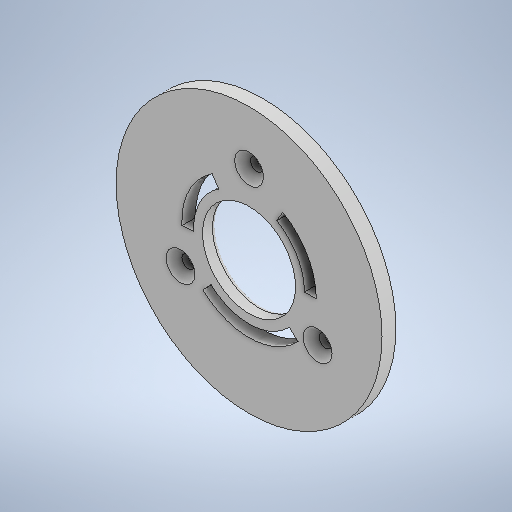
# Autodesk Inventor part: 旋钮帽基座-v0.1.1
Saved by Autodesk Inventor 2025 (Build 290162000, 162)
## iProperties
Created: 2025-05-09
Part Number: 旋钮帽基座-v0.1.1
Material: 常规
Document SubType Name: Modeling
Designer: hawav
Density: 1 g/cm^3
Appearance: 默认
Author: hawav
Autodesk Inventor part; units mm, degrees
ref_plane "YZ Plane" through (0, 0, 0) normal (1, 0, 0) x (0, 1, 0)
ref_plane "XZ Plane" through (0, 0, 0) normal (0, 1, 0) x (-1, 0, 0)
ref_plane "XY Plane" through (0, 0, 0) normal (0, 0, 1) x (1, 0, 0)
sketch "草图1" plane through (0, 0, 0) normal (0, 0, 1) x (1, 0, 0)
  circle A0 centre (0, 0) radius 33.6
  circle A1 centre (0, 0) radius 20
  circle A2 centre (0, 20) radius 1.65
  circle A3 centre (-17.3205, -10) radius 1.65
  circle A4 centre (17.3205, -10) radius 1.65
  circle A5 centre (0, 0) radius 11.75
  circle A6 centre (0, 0) radius 21.65
  line L0 (0, 21.65) -> (0, 33.6)
  circle A7 centre (-5.3894, 27.0942) radius 5.15
  circle A8 centre (-15.3476, 22.9693) radius 5.15
  circle A9 centre (-22.9693, 15.3476) radius 5.15
  circle A10 centre (-27.0942, 5.3894) radius 5.15
  circle A11 centre (-27.0942, -5.3894) radius 5.15
  circle A12 centre (-22.9693, -15.3476) radius 5.15
  circle A13 centre (-15.3476, -22.9693) radius 5.15
  circle A14 centre (-5.3894, -27.0942) radius 5.15
  circle A15 centre (5.3894, -27.0942) radius 5.15
  circle A16 centre (15.3476, -22.9693) radius 5.15
  circle A17 centre (22.9693, -15.3476) radius 5.15
  circle A18 centre (27.0942, -5.3894) radius 5.15
  circle A19 centre (27.0942, 5.3894) radius 5.15
  circle A20 centre (22.9693, 15.3476) radius 5.15
  circle A21 centre (15.3476, 22.9693) radius 5.15
  circle A22 centre (5.3894, 27.0942) radius 5.15
  line L1 (0, 0) -> (0.3894, -13.9946)
  line L2 (0.3894, -13.9946) -> (0.4728, -16.9934)
  arc A23 (0.4728, -16.9934) -> (12.3505, -11.6818) centre (0, 0) ccw
  line L3 (0, 0) -> (12.3505, -11.6818) construction
  line L4 (0, 0) -> (0.4728, -16.9934) construction
  arc A24 (17, 0) -> (8.5, 14.7224) centre (0, 0) ccw
  line L5 (0, 0) -> (8.5, 14.7224) construction
  line L6 (0, 0) -> (17, 0) construction
  arc A25 (0.3894, -13.9946) -> (10.171, -9.6203) centre (0, 0) ccw
  line L7 (0, 0) -> (10.171, -9.6203) construction
  line L8 (0, 0) -> (0.3894, -13.9946) construction
  arc A26 (14, 0) -> (7, 12.1244) centre (0, 0) ccw
  line L9 (7, 12.1244) -> (8.5, 14.7224)
  line L10 (17, 0) -> (14, 0)
  line L11 (12.3505, -11.6818) -> (10.171, -9.6203)
  line L12 (0.4728, -16.9934) -> (0.3894, -13.9946)
  arc A27 (-11.6818, -12.3505) -> (0.4728, -16.9934) centre (0, 0) ccw
  arc A28 (-9.3055, 14.227) -> (-16.9737, -0.9452) centre (0, 0) ccw
  line L13 (0, 0) -> (-9.3055, 14.227) construction
  arc A29 (-9.6203, -10.171) -> (0.3894, -13.9946) centre (0, 0) ccw
  arc A30 (-7.6633, 11.7164) -> (-13.9783, -0.7784) centre (0, 0) ccw
  line L14 (-7.6633, 11.7164) -> (-9.3055, 14.227)
  line L15 (-16.9737, -0.9452) -> (-13.9783, -0.7784)
  line L16 (-11.6818, -12.3505) -> (-9.6203, -10.171)
  dimension "d0" = 67.2
  dimension "d1" = 40
  dimension "d2" = 3.3
  dimension "d10" = 43.3
  dimension "d5" = 360
  dimension "d7" = 23.5
  dimension "d11" = 10.3
  dimension "d14" = 360
  dimension "d18" = 14
  dimension "d19" = 3
  dimension "d20" = 45
  dimension "d21" = 60
  dimension "d22" = 45
  constraints: 34 end point, 27 centre point, 20 point on circle, 11 coincident, 6 symmetric about line, 4 point on line, 4 vertical alignment, 3 collinear, 1 vertical, 52 other
  measures "d7" diameter of A5
  measures "d11" diameter of A7
  measures "d18" distance of L1.start L1.end
  measures "d19" distance of L1.end L2.end
  measures "d20" angle of L4 L3
  measures "d21" angle of L6 L5
  measures "d22" angle of L8 L7
extrude "拉伸1" add sketch "草图1" along normal blind 3.5 contours A0 | A1 A4 A3 A2 | A1 A2 A6 A4 | A1 A3 A6 A2 | A4 A6 A3 A1 | A7 | A8 | A9 | A10 | A11 | A12 | A13 | A14 | A15 | A16 | A17 | A18 | A19 | A20 | A21 | A22 | A25 L11 A23 L2 | L2 A27 L16 A29 | L10 A26 L9 A24 | L14 A30 L15 A28
extrude "拉伸2" cut sketch "草图1" along normal blind 2 contours A7 | A8 | A9 | A10 | A11 | A12 | A13 | A14 | A15 | A16 | A17 | A18 | A19 | A20 | A21 | A22
extrude "拉伸3" cut sketch "草图1" along normal blind 5 contours A25 L11 A23 L2 | L2 A27 L16 A29 | L10 A26 L9 A24 | L14 A30 L15 A28
fillet "圆角1" radius 1 1 edges at (-11.75, 0, 0) curvature continuous yes
chamfer "倒角1" distance 2 angle 45 3 edges at (-18.9705, -10, 3.5) (-1.65, 20, 3.5) (15.6705, -10, 3.5)
